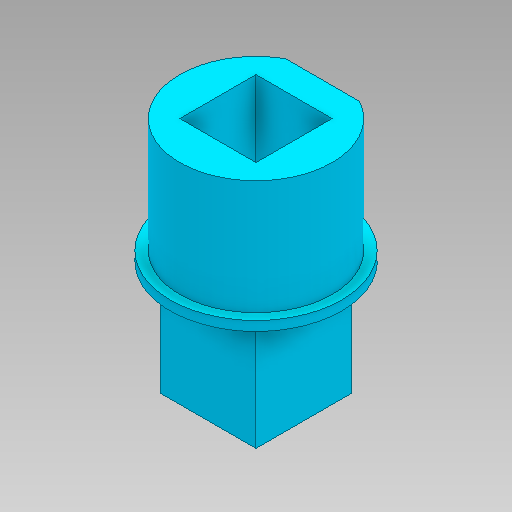
# Autodesk Inventor part: B3-C
Saved by Autodesk Inventor 2018.1 (Build 221171000, 171)
## iProperties
Created: 2018-06-22
Part Number: B3-C
Material: Všeobecné
Document SubType Name: Modeling
Designer: PS
Density: 1 g/cm^3
Appearance: Výchozí
Author: PS
Autodesk Inventor part; units mm, degrees
ref_plane "YZ Plane" through (0, 0, 0) normal (1, 0, 0) x (0, 1, 0)
ref_plane "XZ Plane" through (0, 0, 0) normal (0, 1, 0) x (-1, 0, 0)
ref_plane "XY Plane" through (0, 0, 0) normal (0, 0, 1) x (1, 0, 0)
sketch "Náčrt1" plane through (0, 0, 0) normal (0, 0, 1) x (1, 0, 0)
  line L0 (-200, -200) -> (200, -200)
  line L1 (200, -200) -> (200, 200)
  line L2 (200, 200) -> (-200, 200)
  line L3 (-200, 200) -> (-200, -200)
  line L4 (-200, -200) -> (200, 200) construction
  line L5 (200, -200) -> (-200, 200) construction
  circle A0 centre (0, 0) radius 400
  dimension "d6" = 800
  dimension "d7" = 400
  constraints: 12 end point, 2 parallel, 2 perpendicular, 1 centre point, 1 coincident, 1 horizontal, 1 midpoint
  measures "d6" diameter of A0
  measures "d7" distance of L1.end L2.end
extrude "Vysunutí1" add sketch "Náčrt1" along normal blind 600
sketch "Náčrt2" plane through (0, 0, 0) normal (0, 0, -1) x (-1, 0, 0)
  line L0 (200, 200) -> (200, -200) projected
  line L1 (200, -200) -> (-200, -200) projected
  line L2 (-200, -200) -> (-200, 200) projected
  line L3 (-200, 200) -> (200, 200) projected
  circle A0 centre (0, 0) radius 400 projected
  circle A1 centre (0, 0) radius 450
  dimension "d8" = 900
  constraints: 1 centre point, 1 coincident
  measures "d8" diameter of A1
extrude "Vysunutí2" add sketch "Náčrt2" along normal blind 50 contours A0 | A1
sketch "Náčrt3" plane through (0, 0, 600) normal (0, 0, 1) x (1, 0, 0)
  line L0 (251.7841, 450) -> (-248.2159, 450)
  line L1 (-248.2159, 450) -> (-248.2159, 350)
  line L2 (-248.2159, 350) -> (251.7841, 350)
  line L3 (251.7841, 350) -> (251.7841, 450)
  circle A0 centre (0, 0) radius 400 projected
  dimension "d11" = 350
  dimension "d12" = 100
  dimension "d13" = 500
  constraints: 8 end point, 2 parallel, 1 horizontal, 1 perpendicular
  measures "d11" distance from line of L2 A0.centre
  measures "d12" distance of L2.end L0.start
  measures "d13" distance of L0.start L0.end
extrude "Vysunutí3" cut sketch "Náčrt3" against normal blind 50 contours L3 L2 A0 L1 L0 | L2 A0 picked at (-56.548, 354.0814)
sketch "Náčrt4" plane through (0, 0, -50) normal (0, 0, -1) x (-1, 0, 0)
  line L0 (200, -200) -> (-200, -200) projected
  line L1 (200, 200) -> (200, -200) projected
  line L2 (-200, 200) -> (200, 200) projected
  line L3 (-200, -200) -> (-200, 200) projected
  line L4 (-250, -250) -> (250, -250)
  line L5 (250, -250) -> (250, 250)
  line L6 (250, 250) -> (-250, 250)
  line L7 (-250, 250) -> (-250, -250)
  point P0 (0, 0)
  dimension "d16" = 50
  constraints: 8 end point, 3 other
  measures "d16" distance between parallel lines of L0 L4
extrude "Vysunutí4" add sketch "Náčrt4" along normal blind 600
